ansi41sprocket1001 (Autodesk Fusion 360 design; units mm, degrees)
Autodesk Fusion 360 part; units mm, degrees
note: some values were not read from the file. Set by a fixed rule: which sketch regions a step uses.
sketch "Sketch1" plane through (0, 0, 0) normal (0, 0, 1) x (1, 0, 0)
  line L0 (-2.8829, 0) -> (0, 0)
  line L1 (-2.8829, 0) -> (-2.8829, 10.668)
  line L2 (-2.8829, 10.668) -> (-1.2954, 17.018)
  line L3 (-1.2954, 17.018) -> (0, 17.018)
  line L4 (0, 150) -> (0, -70) construction
  line L5 (-20.32, 7.3176) -> (20.32, 7.3176) construction
  line L6 (2.8829, 0) -> (2.8829, 10.668)
  line L7 (2.8829, 0) -> (-2.8829, 0)
  line L8 (2.8829, 10.668) -> (1.2954, 17.018)
  line L9 (1.2954, 17.018) -> (0, 17.018)
  line L10 (2.8829, 0) -> (-19.3421, 0) construction
  dimension "d7" = 6.35
  dimension "d8" = 1.5875
  dimension "d10" = 5.7658
  dimension "d11" = 22.225
  dimension "d12" = 17.018
  dimension "d56" = 7.3176
  measures "d7" distance of L1.end L3
  measures "d8" distance of L1.end L2.end
  measures "d10" distance of L1 L6
  measures "d11" distance of L6.start L10.end
  measures "d12" distance of L9 L10
  measures "d25" distance of L1.end
  measures "d38" angle of L1.end
  measures "d39" angle of L1.end
  measures "d56" distance of L5 L10
sketch "Sketch2" plane through (0, 0, 0) normal (1, 0, 0) x (0, 0, -1)
  circle A0 centre (0, 0) radius 14.6353 construction
  circle A1 centre (0, 0) radius 16.4845 construction
  circle A2 centre (0, 0) radius 29.9909 construction
  line L0 (0, 0) -> (14.6353, 0) construction
  line L1 (14.6353, 0) -> (7.3176, -12.6745) construction
  line L2 (0, 0) -> (7.3176, -12.6745) construction
  circle A3 centre (7.3176, -12.6745) radius 3.8862 construction
  circle A4 centre (7.3176, -12.6745) radius 3.9262 construction
  line L3 (0, 27.94) -> (0, -29.9909) construction
  line L4 (-1.7689, -17.9206) -> (9.869, -11.2015) construction
  arc A5 (8.428, -8.9086) -> (5.3545, -9.2743) centre (7.3176, -12.6745) ccw
  line L5 (7.3176, -12.6745) -> (-11.7452, -12.6745) construction
  line L6 (-11.8689, -16.4845) -> (10.16, -16.4845) construction
  line L7 (8.428, -8.9086) -> (0, -37.492) construction
  arc A6 (5.3545, -9.2743) -> (3.501, -11.7532) centre (7.3176, -12.6745) ccw
  circle A7 centre (7.3176, -12.6745) radius 3.8862 construction
  line L8 (0, -9.01) -> (7.2659, -21.5949) construction
  line L9 (37.842, 0) -> (4.2401, -19.4001) construction
  line L10 (5.5591, -18.6386) -> (14.8229, 0) construction
  arc A8 (10.0741, -9.5546) -> (8.428, -8.9086) centre (5.5591, -18.6386) ccw
  line L11 (10.0741, -9.5546) -> (26.0323, -17.4862) construction
  line L12 (12.7583, -3.251) -> (234.3352, -121.0182)
  line L13 (10.0741, -9.5546) -> (234.3352, -121.0182)
  point P0 (12.7583, -3.251)
  point P1 (-3.5637, -12.6745)
  dimension "d13" = 14.6353
  dimension "d15" = 7.7724
  dimension "d16" = 7.8525
  dimension "d17" = 3.9262
  dimension "d18" = 3.81
  dimension "d23" = 10.8814
  dimension "d24" = 43.571
  dimension "d25" = 4.505
  dimension "d26" = 4.2858
  dimension "d27" = 10
  measures "d13" distance of L0.end L1.end
  measures "d15" diameter of A3
  measures "d16" diameter of A4
  measures "d17" radius of A5
  measures "d18" distance of L5 L6
  measures "d23" distance of L1.end P0
  measures "d24" angle of L4 L7
  measures "d25" distance of L2 L8
  measures "d26" distance of L4 L9
  measures "d27" angle of L7 L10
sketch "Sketch3" plane through (0, 0, 0) normal (1, 0, 0) x (0, 0, -1)
  circle A0 centre (0, 0) radius 14.6353 construction
  circle A1 centre (0, 0) radius 18.4453 construction
  circle A2 centre (3.1411, -14.2942) radius 3.9437 construction
  circle A3 centre (3.1411, -14.2942) radius 3.8862 construction
  line L0 (3.1411, -14.2942) -> (13.1341, -6.4565) construction
  line L1 (-18.2745, 67.4711) -> (13.1341, -6.4565) construction
  line L2 (0, 0) -> (3.216, -14.6353) construction
  line L3 (-0.8677, -17.0412) -> (-0.3391, -19.447) construction
  line L4 (0, 0) -> (0, -85.9346) construction
  line L5 (9.9049, -12.8079) -> (51.6776, -3.6285) construction
  line L6 (-0.3391, -19.447) -> (46.5173, -9.1505) construction
  line L7 (-0.3391, -19.447) -> (-2.2237, -22.2374) construction
  arc A4 (6.7243, -12.1416) -> (5.3484, -11.0261) centre (-0.3391, -19.447) ccw
  line L8 (-0.3391, -19.447) -> (83.6995, 67.4711) construction
  line L9 (24.8551, -67.4297) -> (11.7031, -7.5788) construction
  line L10 (11.7031, -7.5788) -> (50.6506, 0.9797) construction
  line L11 (6.7243, -12.1416) -> (7.0174, -12.4251)
  line L12 (11.7031, -7.5788) -> (7.0174, -12.4251) construction
  line L13 (-1.0144, -13.8422) -> (-1.1618, -14.2224)
  arc A5 (-0.233, -12.2525) -> (-1.0144, -13.8422) centre (8.4609, -17.5132) ccw
  line L14 (-35.56, -14.6353) -> (40.64, -14.6353) construction
  line L15 (-43.18, -18.4453) -> (38.1, -18.4453) construction
  arc A6 (5.3484, -11.0261) -> (-0.233, -12.2525) centre (3.1411, -14.2942) ccw
  arc A7 (7.0174, -12.4251) -> (11.2176, -14.3024) centre (11.7031, -7.5788) ccw
  line L16 (0, 0) -> (11.3834, -14.5137) construction
  line L17 (12.9605, -16.5244) -> (73.0742, -93.1688) construction
  arc A8 (-4.188, -17.6877) -> (-1.1618, -14.2224) centre (-7.4475, -11.7871) ccw
  arc A9 (11.2176, -14.3024) -> (10.3952, -9.7758) centre (4.5721, -13.1718) ccw
  line L18 (10.1897, -9.4236) -> (10.3952, -9.7758)
  arc A10 (9.4341, -7.8215) -> (10.1897, -9.4236) centre (18.9677, -4.3043) ccw
  arc A11 (11.9552, -2.6931) -> (9.4341, -7.8215) centre (13.1341, -6.4565) ccw
  arc A12 (13.6852, -2.3129) -> (11.9552, -2.6931) centre (14.9928, -12.3901) ccw
  line L19 (13.6852, -2.3129) -> (14.0896, -2.2604)
  arc A13 (14.0896, -2.2604) -> (18.1761, -0.1471) centre (13.2221, 4.4245) ccw
  arc A14 (18.1761, -0.1471) -> (14.1243, 2.0321) centre (13.1488, -4.6379) ccw
  line L20 (13.7208, 2.0912) -> (14.1243, 2.0321)
  arc A15 (11.9972, 2.4993) -> (13.7208, 2.0912) centre (15.1914, 12.1458) ccw
  arc A16 (9.5595, 7.6678) -> (11.9972, 2.4993) centre (13.2369, 6.2431) ccw
  arc A17 (10.3409, 9.2574) -> (9.5595, 7.6678) centre (19.0348, 3.9968) ccw
  line L21 (10.3409, 9.2574) -> (10.552, 9.6063)
  arc A18 (10.552, 9.6063) -> (11.4476, 14.119) centre (4.7846, 13.0961) ccw
  arc A19 (11.4476, 14.119) -> (7.2176, 12.3099) centre (11.8242, 7.3885) ccw
  line L22 (6.9199, 12.0312) -> (7.2176, 12.3099)
  arc A20 (5.5261, 10.9381) -> (6.9199, 12.0312) centre (-0.0243, 19.4499) ccw
  arc A21 (-0.0347, 12.2547) -> (5.5261, 10.9381) centre (3.372, 14.2415) ccw
  arc A22 (-0.7903, 13.8568) -> (-0.0347, 12.2547) centre (8.7432, 17.374) ccw
  line L23 (-0.7903, 13.8568) -> (-0.9315, 14.2393)
  arc A23 (-0.9315, 14.2393) -> (-3.9012, 17.7531) centre (-7.2558, 11.9061) ccw
  arc A24 (-3.9012, 17.7531) -> (-5.1242, 13.318) centre (1.5957, 13.8512) ccw
  line L24 (-5.0919, 12.9115) -> (-5.1242, 13.318)
  arc A25 (-5.1062, 11.1403) -> (-5.0919, 12.9115) centre (-15.2217, 12.1078) ccw
  arc A26 (-9.6028, 7.6135) -> (-5.1062, 11.1403) centre (-9.0321, 11.5158) ccw
  arc A27 (-11.3264, 8.0217) -> (-9.6028, 7.6135) centre (-8.1322, 17.6682) ccw
  line L25 (-11.3264, 8.0217) -> (-11.7135, 8.1498)
  arc A28 (-11.7135, 8.1498) -> (-16.3123, 8.0188) centre (-13.8325, 1.7505) ccw
  arc A29 (-16.3123, 8.0188) -> (-13.6073, 4.2974) centre (-9.8344, 9.8837) ccw
  line L26 (-13.2694, 4.0692) -> (-13.6073, 4.2974)
  arc A30 (-11.8935, 2.9536) -> (-13.2694, 4.0692) centre (-18.9568, -4.3517) ccw
  arc A31 (-11.9397, -2.7608) -> (-11.8935, 2.9536) centre (-14.6348, 0.1184) ccw
  arc A32 (-13.3335, -3.8539) -> (-11.9397, -2.7608) centre (-18.8839, 4.6579) ccw
  line L27 (-13.3335, -3.8539) -> (-13.6751, -4.0767)
  arc A33 (-13.6751, -4.0767) -> (-16.4399, -7.7538) centre (-9.993, -9.7232) ccw
  circle A34 centre (0, 0) radius 18.1767
  arc A35 (-16.4399, -7.7538) -> (-11.8439, -7.9592) centre (-13.859, -1.5264) ccw
  line L28 (-11.4547, -7.8373) -> (-11.8439, -7.9592)
  arc A36 (-9.7247, -7.4572) -> (-11.4547, -7.8373) centre (-8.4171, -17.5343) ccw
  arc A37 (-5.2858, -11.0562) -> (-9.7247, -7.4572) centre (-9.2172, -11.3681) ccw
  arc A38 (-5.3002, -12.8274) -> (-5.2858, -11.0562) centre (-15.4157, -11.8599) ccw
  line L29 (-5.3002, -12.8274) -> (-5.339, -13.2334)
  arc A39 (-5.339, -13.2334) -> (-4.188, -17.6877) centre (1.3714, -13.8752) ccw
  point P0 (-7.4475, -11.7871)
  dimension "d28" = 7.7724
  dimension "d29" = 7.8875
  dimension "d30" = 12.7
  dimension "d31" = 4.505
  dimension "d37" = 4.2858
  dimension "d38" = 36.5
  dimension "d39" = 10
  dimension "d40" = 9.8038
  dimension "d41" = 4.7212
  dimension "d42" = 3.81
  dimension "d43" = 3.9437
  dimension "d45" = 25.714
  dimension "d47" = 360
  measures "d28" diameter of A3
  measures "d29" diameter of A2
  measures "d30" distance of A2.centre L0.end
  measures "d31" distance of L2 L3
  measures "d37" distance of L5 L6
  measures "d39" angle of L7 L8
  measures "d40" distance of L2 L9
  measures "d41" distance of L5 L10
  measures "d42" distance of L14 L15
  measures "d43" radius of A6
  measures "d45" angle of L2 L16
revolve "Revolve1" add sketch "Sketch1" angle 360 about axis through (2.8829, 0, 0) along (-1, 0, 0)
extrude "Extrude1" cut sketch "Sketch3" along normal mid plane 10.16 contours A4 L11 L13 A5 A6 A7 A8 A34
pattern_circular "C-Pattern1" count 7 over 360 about axis through (2.8829, 0, 0) along (-1, 0, 0) of "Extrude1"
sketch "Sketch4" plane through (-2.8829, 0, 0) normal (-1, 0, 0) x (0, 0, 1)
  circle A0 centre (0, 0) radius 9.525
  circle A1 centre (0, 0) radius 10.668
  dimension "d53" = 19.05
  measures "d53" diameter of A0
extrude "Extrude2" add sketch "Sketch4" along normal up to surface (16.4592 mm away) contours A0
sketch "Sketch5" plane through (0, 0, 0) normal (0, 0, 1) x (1, 0, 0)
  line L0 (-2.8829, 12.065) -> (-2.8829, 7.3176)
  line L1 (-2.8829, 7.3176) -> (-6.4865, 7.3176)
  line L2 (-6.4865, 7.3176) -> (-6.4865, 12.065)
  line L3 (-6.4865, 12.065) -> (-2.8829, 12.065)
  line L4 (-20.32, 7.3176) -> (20.32, 7.3176)
  line L5 (2.8829, 0) -> (-19.3421, 0)
  line L6 (-18.7071, 9.525) -> (-19.3421, 9.525)
  line L7 (-19.3421, 9.525) -> (-19.3421, 8.89)
  line L8 (-19.3421, 8.89) -> (-18.7071, 9.525)
  line L9 (-2.8829, -10.668) -> (-2.8829, 10.668)
  point P0 (-19.3421, 0)
  dimension "d57" = 12.065
  dimension "d58" = 3.6036
  dimension "d59" = 9.525
  dimension "d60" = 0.635
  measures "d57" distance of L3 L5
  measures "d58" distance of L0.start L2.end
  measures "d59" distance of L6 P0
  measures "d60" distance of L6.start L6.end
revolve "Revolve2" cut sketch "Sketch5" angle 360 about axis through (2.8829, 0, 0) along (-1, 0, 0)
sketch "Sketch6" plane through (2.8829, 0, 0) normal (1, 0, 0) x (0, 0, -1)
  circle A0 centre (0, 0) radius 4.7625
  circle A1 centre (0, 0) radius 10.668
  dimension "d62" = 9.525
  measures "d62" diameter of A0
extrude "Extrude3" cut sketch "Sketch6" against normal up to surface (22.225 mm away) contours A0
equation "No_teeth = 7"
equation "Innershaft_dia = ( 3 / 8 ) * 1 in"
equation "OD = 1.34 in"
equation "Overall_width = ( 7 / 8 ) * 1 in"
equation "Hub_dia = ( 3 / 4 ) * 1 in"
equation "Gear_thickness = 0.227 in"
equation "d7 = Tooth_pitch / 2"
equation "d8 = d7 / 4"
equation "d10 = Gear_thickness"
equation "d11 = Overall_width"
equation "d12 = OD / 2"
equation "d13 = Tooth_pitch / sin(( 180 / No_teeth ) * 1 deg) / 2"
equation "Tooth_pitch = 0.5 in"
equation "d16 = 1.0005 * d15 + 0.003 in"
equation "d17 = d16 / 2"
equation "d23 = 1.4 * d15"
equation "d24 = 35 deg + ( ( 60 / No_teeth ) * 1 deg )"
equation "d25 = 0.8 * d15 * cos(35 deg + ( ( 60 / No_teeth ) * 1 deg ))"
equation "d26 = 0.8 * d15 * sin(35 deg + ( ( 60 / No_teeth ) * 1 deg ))"
equation "d27 = 18 deg - ( ( 56 / No_teeth ) * 1 deg )"
equation "d29 = 1.005 * d28 + 0.003 in"
equation "d30 = Tooth_pitch"
equation "d31 = 0.8 * d28 * cos(35 deg + ( ( 60 / No_teeth ) * 1 deg ))"
equation "d37 = 0.8 * d28 * sin(35 deg + ( ( 60 / No_teeth ) * 1 deg ))"
equation "d39 = 18 deg - ( ( 56 / No_teeth ) * 1 deg )"
equation "d40 = 1.4 * d28 * cos(( 180 / No_teeth ) * 1 deg)"
equation "d41 = 1.4 * d28 * sin(( 180 / No_teeth ) * 1 deg)"
equation "d42 = 0.3 * d30"
equation "d43 = d29 / 2"
equation "d45 = ( 180 / No_teeth ) * 1 deg"
equation "d46 = No_teeth"
equation "d51 = No_teeth"
equation "d53 = Hub_dia"
equation "d56 = pitch_cir_dia / 4"
equation "d57 = Hub_dia / 2 + 0.1 in"
equation "d58 = Gear_thickness * 5 / 8"
equation "d59 = Hub_dia / 2"
equation "d62 = Innershaft_dia"
equation "pitch_cir_dia = ( 0.5 / sin(( 180 / No_teeth ) * 1 deg) ) * 1 in"
